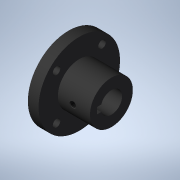
# Autodesk Inventor part: STHRANG10-MB_ss
Saved by Autodesk Inventor 2021 (Build 250183000, 183)
## iProperties
Created: 2025-08-06
Part Number: STHRANG10-MB_ss
Material: Generic
Catalog Web Link: www.cadenas.de
Description: STHRBNG, STHRNG, SSTHRNG, STHRANG_SS-Shaft Supports - with Damper - Key Groove - Round Flange
Vendor: MISUMI
Document SubType Name: Modeling
Designer: psAdmin
Manufacturer: MISUMI
Mass: 8.46774 g
Surface Area: 45.3297 cm^2
Volume: 8.46774 cm^3
Density: 1 g/cm^3
Appearance: PSOLRGB-175-175-175
Category: PARTsolutions
Company: MISUMI
Title: STHRANG10-MB
Author: Cadenas PARTsolutions
Comments: Shaft Supports - with Damper - Key Groove - Round Flange
PSOL_IDENT_0: {$CADENAS_DATA/23d-libs/misumi/metric/02_shaft_supports/sthrbng/sthrbng.prj},209 {VTYP=3D},{NB=STHRA
PSOL_IDENT_1: NG10-MB_ss},{LINA=STHRANG10-MB},{NN=STHRBNG, STHRNG, SSTHRNG, STHRANG_SS},{DATE=18.02.2024 15:03:40}
PSOL_IDENT_2: ,{GEOMDATE=16.02.2024 10:05:26},{VERSION=},{LINEID=200},{WBVAR=MAT,ST,ALT1},{WBNUMERIC=}  {NB=STHRAN
PSOL_IDENT_3: G10-MB_ss},{LINA=STHRANG10-MB},{KT=DUMMY},{PN=STHRANG10-MB},{TYPE=STHRANG},{MAT=5052},{ST=-},{D=10},
PSOL_IDENT_4: {DTOL=+0.015/0},{N=5.0},{L=20},{S=0},{L1=0},{D1=20},{H=38},{T=5},{LL=12},{M=M3},{THMD=3},{THDMIN=2.4
PSOL_IDENT_5: 59},{P=30},{K=0},{W=20},{P1=30},{F=0},{DD1=3.5},{ST0='-','-'},{BB=3},{BBTOL=+0.013/-0.013},{TT=1.8},
PSOL_IDENT_6: {TTTOL=+0.1/0},{ALT1=MB},{MBM=M3},{ML=3},{ALT1PN=-MB},{MATALG= '1045', 'S45C Equivalent', '304', 'SU
PSOL_IDENT_7: S304','5052','5052 Aluminum Alloy' }
NB: STHRANG10-MB_ss
NN: STHRBNG, STHRNG, SSTHRNG, STHRANG_SS
NT: Shaft Supports - with Damper - Key Groove - Round Flange
NBSYN: $PN._ss
LINA: STHRANG10-MB
CATALOG: Misumi
PN: STHRANG10-MB
MAT: 5052 Aluminum Alloy
ST: -
D: 10
DTOL: +0.015/0
N: 5
L: 20
S: 0
L1: 0
D1: 20
H: 38
T: 5
LL: 12
M: M3
P: 30
W: 20
P1: 30
F: 0
DD1: 3.5
BB: 3
BBTOL: +0.013/-0.013
TT: 1.8
TTTOL: +0.1/0
MBM: M3
ML: 3
SUPPLIER: MISUMI
ARTICLENO: STHRANG10-MB_ss
BOMINFO: STHRANG10-MB
CREATOR: CADENAS GmbH
Autodesk Inventor part; units mm, degrees
sketch "Sketch_1" plane through (0, 0, 0) normal (0, 0, 1) x (1, 0, 0)
  line L0 (20, 0) -> (0, 0)
  line L1 (0, 5) -> (20, 5)
  line L2 (20, 5) -> (20, 10)
  line L3 (20, 10) -> (5, 10)
  line L4 (5, 10) -> (5, 19)
  line L5 (5, 19) -> (0, 19)
  line L6 (0, 19) -> (0, 5)
  constraints: 14 end point
revolve "Revolution1" add sketch "Sketch_1" angle 360 about axis through (20, 0, 0) along (1, 0, 0)
sketch "Sketch2" plane through (0, 0, 0) normal (-1, 0, 0) x (0, 0, 1)
  point P0 (-10.6066, 10.6066)
hole "Hole1" at (0, 10.6066, -10.6066) direction (1, 0, 0) diameter 3.5 depth 5
pattern_linear "Rectangular Pattern1" count 2 spacing 21.2132 along (0, 0, 1) count 2 spacing 21.2132 along (0, -1, 0) of "Hole1"
sketch "Sketch_4" plane through (12, 0, 0) normal (1, 0, 0) x (0, 0, -1)
  line L0 (0, -10) -> (0, -4)
  line L1 (0, -4) -> (1.2295, -4)
  line L2 (1.2295, -4) -> (1.2295, -9.7295)
  line L3 (1.2295, -9.7295) -> (1.5, -10)
  line L4 (1.5, -10) -> (0, -10)
  line L5 (0, -10) -> (0, -4)
  constraints: 12 end point
revolve "Revolution2" cut sketch "Sketch_4" angle 360 about axis through (12, -10, 0) along (0, -1, 0)
thread "Thread1" size "M3x0.5" class "6H" standard "ISO Metric profile" full length
sketch "Sketch_8" plane through (0, 0, 0) normal (1, 0, 0) x (0, 1, 0)
  line L0 (1.5, 6.8) -> (-1.5, 6.8)
  line L1 (-1.5, 6.8) -> (-1.5, 0)
  line L2 (-1.5, 0) -> (1.5, 0)
  line L3 (1.5, 0) -> (1.5, 6.8)
  constraints: 8 end point
extrude "Extrusion1" cut sketch "Sketch_8" along normal blind 20
sketch "Sketch_5" plane through (12, 0, 0) normal (1, 0, 0) x (0, 0, -1)
  line L0 (-5, 0) -> (-10, 0)
  line L1 (-10, 0) -> (-10, 1.5)
  line L2 (-10, 1.5) -> (-9.7295, 1.2295)
  line L3 (-9.7295, 1.2295) -> (-5, 1.2295)
  line L4 (-5, 1.2295) -> (-5, 0)
  line L5 (-5, 0) -> (-10, 0)
  constraints: 12 end point
revolve "Revolution3" cut sketch "Sketch_5" angle 360 about axis through (12, 0, 5) along (0, 0, -1)
thread "Thread2" size "M3x0.5" class "6H" standard "ISO Metric profile" length 2.9295
ref_plane "to_screw1_XY" through (12, 0, 6.8) normal (0, 0, 1) x (1, 0, 0)
ref_plane "to_screw1_YZ" through (12, 0, 6.8) normal (1, 0, 0) x (0, 1, 0)
ref_plane "to_screw1_ZX" through (12, 0, 6.8) normal (0, 1, 0) x (0, 0, 1)
ref_plane "to_screw2_XY" through (12, -5, 0) normal (0, -1, 0) x (1, 0, 0)
ref_plane "to_screw2_YZ" through (12, -5, 0) normal (1, 0, 0) x (0, 0, 1)
ref_plane "to_screw2_ZX" through (12, -5, 0) normal (0, 0, 1) x (0, -1, 0)
body "Solid1"
